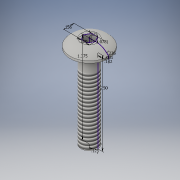
# Autodesk Inventor part: Sun_AxlePeg
Saved by Autodesk Inventor 2016 (Build 200138000, 138)
## iProperties
Created: 2018-01-10
Part Number: Sun_AxlePeg
Material: Generic
Document SubType Name: Modeling
Designer: sun01147
Density: 1 g/cm^3
Appearance: Default
Author: sun01147
Autodesk Inventor part; units mm, degrees
ref_plane "YZ Plane" through (0, 0, 0) normal (1, 0, 0) x (0, 1, 0)
ref_plane "XZ Plane" through (0, 0, 0) normal (0, 1, 0) x (-1, 0, 0)
ref_plane "XY Plane" through (0, 0, 0) normal (0, 0, 1) x (1, 0, 0)
sketch "Sketch1" plane through (0, 0, 0) normal (0, 0, 1) x (1, 0, 0)
  line L0 (0, 0) -> (0, 34.925)
  line L1 (0, 0) -> (3.175, 0)
  line L2 (3.175, 0) -> (3.175, 31.75)
  line L3 (3.175, 31.75) -> (7.2796, 31.75)
  line L4 (0, 34.925) -> (3.175, 34.925)
  line L5 (7.2796, 31.75) -> (7.2796, 32.5374)
  arc A0 (7.2796, 32.5374) -> (3.175, 34.925) centre (2.4597, 28.9734) ccw
  dimension "d1" = 3.175
  dimension "d2" = 31.75
  dimension "d3" = 34.925
  dimension "d6" = 3.175
  dimension "d9" = 4.1046
  dimension "d10" = 5.9944
  dimension "d11" = 0.7874
  constraints: 12 end point, 3 horizontal, 3 vertical, 2 point on circle, 1 centre point
  measures "d1" distance of L0.start L1.end
  measures "d2" distance of L1.end L2.end
  measures "d3" distance of L0.start L0.end
  measures "d6" distance of L0.end L4.end
  measures "d9" distance of L2.end L3.end
  measures "d10" radius of A0
  measures "d11" distance of L3.end L5.end
revolve "Revolution1" add sketch "Sketch1" angle 360 about axis through (0, 0, 0) along (0, 1, 0)
sketch "Sketch2" plane through (0, 34.925, 0) normal (0, 1, 0) x (1, 0, 0)
  line L0 (1.1539, -1.9796) -> (-1.1374, -1.9891)
  line L1 (-1.1374, -1.9891) -> (-2.2913, -0.0095)
  line L2 (-2.2913, -0.0095) -> (-1.1539, 1.9796)
  line L3 (-1.1539, 1.9796) -> (1.1374, 1.9891)
  line L4 (1.1374, 1.9891) -> (2.2913, 0.0095)
  line L5 (2.2913, 0.0095) -> (1.1539, -1.9796)
  point P0 (0, 0)
  point P1 (0, 0)
  dimension "d13" = 3.9688
  dimension "d14" = 1.9844
  dimension "d15" = 4.5827
  constraints: 12 end point, 1 coincident, 13 other
  measures "d13" distance between parallel lines of L0 L3
  measures "d14" distance from line of L3 point (0, 0)
  measures "d15" horizontal distance of L4.end L1.end
sketch "Sketch3" plane through (0, 34.925, 0) normal (0, 1, 0) x (1, 0, 0)
  point P0 (0, 0)
extrude "Extrusion1" cut sketch "Sketch2" against normal blind 2.8194
thread "Thread1" size "1/4-20 UNC" class "2A" standard "ANSI Unified Screw Threads" length 25.4
body "Solid1"
